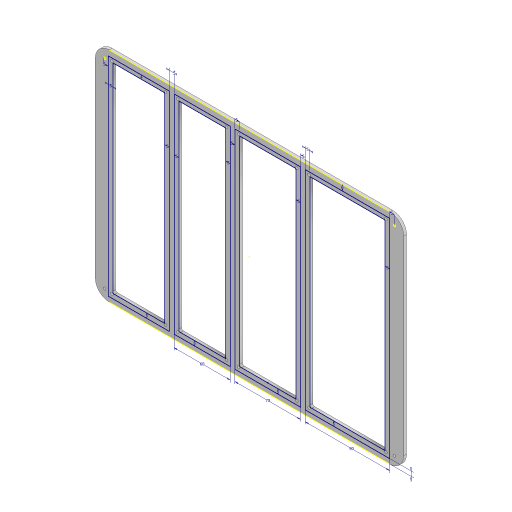
# Autodesk Inventor part: рамка насу
Saved by Autodesk Inventor 2023.2 (Build 272271000, 271)
## iProperties
Created: 2023-02-13
Part Number: рамка насу
Material: Типовые
Document SubType Name: Modeling
Designer: User
Density: 1 g/cm^3
Appearance: По умолчанию
Author: User
Autodesk Inventor part; units mm, degrees
ref_plane "YZ Plane" through (0, 0, 0) normal (1, 0, 0) x (0, 1, 0)
ref_plane "XZ Plane" through (0, 0, 0) normal (0, 1, 0) x (-1, 0, 0)
ref_plane "XY Plane" through (0, 0, 0) normal (0, 0, 1) x (1, 0, 0)
sketch "Эскиз1" plane through (0, 0, 0) normal (0, 0, 1) x (1, 0, 0)
  line L0 (-149.5, 116.5) -> (149.5, 116.5)
  line L1 (164.5, 101.5) -> (164.5, -101.5)
  line L2 (149.5, -116.5) -> (-149.5, -116.5)
  line L3 (-164.5, -101.5) -> (-164.5, 101.5)
  line L4 (0, -167.4492) -> (0, 167.4492) projected
  line L5 (-234.6492, 0) -> (234.6492, 0) projected
  arc A0 (-149.5, 116.5) -> (-164.5, 101.5) centre (-149.5, 101.5) ccw
  arc A1 (164.5, 101.5) -> (149.5, 116.5) centre (149.5, 101.5) ccw
  arc A2 (149.5, -116.5) -> (164.5, -101.5) centre (149.5, -101.5) ccw
  arc A3 (-164.5, -101.5) -> (-149.5, -116.5) centre (-149.5, -101.5) ccw
  circle A4 centre (-154.5, 106.5) radius 1.35
  circle A5 centre (154.5, 106.5) radius 1.35
  circle A6 centre (154.5, -106.5) radius 1.35
  circle A7 centre (-154.5, -106.5) radius 1.35
  point P0 (0, 0)
  dimension "d0" = 329
  dimension "d1" = 233
  dimension "d2" = 15
  dimension "d3" = 2.7
  dimension "d4" = 2.7
  dimension "d5" = 2.7
  dimension "d6" = 2.7
  dimension "d7" = 5
  dimension "d8" = 5
  dimension "d9" = 5
  dimension "d10" = 5
  dimension "d11" = 5
  dimension "d12" = 5
  dimension "d13" = 5
  dimension "d14" = 5
  constraints: 8 centre point, 8 end point, 8 point on circle, 8 tangent, 3 equal radius, 2 parallel, 1 horizontal, 1 perpendicular, 2 other
  measures "d0" distance between parallel lines of L1 L3
  measures "d1" distance between parallel lines of L2 L0
  measures "d2" radius of A0
  measures "d3" diameter of A4
  measures "d4" diameter of A5
  measures "d5" diameter of A6
  measures "d6" diameter of A7
  measures "d7" horizontal distance of A6.centre A2.centre
  measures "d8" horizontal distance of A2.centre A6.centre
  measures "d9" horizontal distance of A1.centre A5.centre
  measures "d10" horizontal distance of A5.centre A1.centre
  measures "d11" horizontal distance of A0.centre A4.centre
  measures "d12" horizontal distance of A0.centre A4.centre
  measures "d13" horizontal distance of A7.centre A3.centre
  measures "d14" horizontal distance of A3.centre A7.centre
extrude "Выдавливание1" add sketch "Эскиз1" along normal blind 3
sketch "Эскиз2" plane through (0, 0, 3) normal (0, 0, 1) x (1, 0, 0)
  line L0 (149.5, 110.5) -> (59.5, 110.5)
  line L1 (59.5, 110.5) -> (59.5, -111.5)
  line L2 (59.5, -111.5) -> (149.5, -111.5)
  line L3 (149.5, -111.5) -> (149.5, 110.5)
  line L4 (54.5, 110.5) -> (-15.5, 110.5)
  line L5 (-15.5, 110.5) -> (-15.5, -111.5)
  line L6 (-15.5, -111.5) -> (54.5, -111.5)
  line L7 (54.5, -111.5) -> (54.5, 110.5)
  line L8 (-20.5, 110.5) -> (-80.5, 110.5)
  line L9 (-80.5, 110.5) -> (-80.5, -111.5)
  line L10 (-80.5, -111.5) -> (-20.5, -111.5)
  line L11 (-20.5, -111.5) -> (-20.5, 110.5)
  circle A0 centre (154.5, 106.5) radius 1.35 projected
  line L12 (-85.5, 110.5) -> (-150.85, 110.5)
  line L13 (-150.85, 110.5) -> (-150.85, -111.5)
  line L14 (-150.85, -111.5) -> (-85.5, -111.5)
  line L15 (-85.5, -111.5) -> (-85.5, 110.5)
  circle A1 centre (-154.5, 106.5) radius 1.35 projected
  line L16 (-149.5, -116.5) -> (149.5, -116.5) projected
  line L17 (149.5, 116.5) -> (-149.5, 116.5) projected
  line L18 (-145.85, 106.5) -> (-90.5, 106.5)
  line L19 (-90.5, 106.5) -> (-90.5, -106.5)
  line L20 (-90.5, -106.5) -> (-145.85, -106.5)
  line L21 (-145.85, -106.5) -> (-145.85, 106.5)
  line L22 (-75.5, 106.5) -> (-25.5, 106.5)
  line L23 (-25.5, 106.5) -> (-25.5, -106.5)
  line L24 (-25.5, -106.5) -> (-75.5, -106.5)
  line L25 (-75.5, -106.5) -> (-75.5, 106.5)
  line L26 (-10.5, 106.5) -> (49.5, 106.5)
  line L27 (49.5, 106.5) -> (49.5, -106.5)
  line L28 (49.5, -106.5) -> (-10.5, -106.5)
  line L29 (-10.5, -106.5) -> (-10.5, 106.5)
  line L30 (64.5, 106.5) -> (144.5, 106.5)
  line L31 (144.5, 106.5) -> (144.5, -106.5)
  line L32 (144.5, -106.5) -> (64.5, -106.5)
  line L33 (64.5, -106.5) -> (64.5, 106.5)
  point P0 (0, 0)
  point P1 (19.5, -106.5)
  dimension "d18" = 70
  dimension "d19" = 60
  dimension "d20" = 5
  dimension "d21" = 5
  dimension "d22" = 5
  dimension "d23" = 90
  dimension "d25" = 5
  dimension "d26" = 5
  dimension "d27" = 5
  dimension "d29" = 6
  dimension "d30" = 4
  dimension "d31" = 5
  dimension "d32" = 5
  dimension "d33" = 5
  dimension "d34" = 5
  dimension "d35" = 5
  dimension "d36" = 5
  dimension "d37" = 5
  dimension "d38" = 5
  dimension "d39" = 5
  dimension "d40" = 5
  dimension "d41" = 5
  dimension "d42" = 5
  constraints: 64 end point, 16 parallel, 8 horizontal, 8 perpendicular, 5 horizontal alignment, 4 point on line, 1 midpoint
  measures "d18" distance of L6.end L5.end
  measures "d19" distance of L10.end L9.end
  measures "d20" distance between parallel lines of L7 L1
  measures "d21" distance from line of A0.centre L3
  measures "d22" distance between parallel lines of L11 L5
  measures "d23" distance between parallel lines of L3 L1
  measures "d25" distance between parallel lines of L15 L9
  measures "d27" distance between parallel lines of L2 L16
  measures "d29" distance between parallel lines of L17 L0
  measures "d30" distance between parallel lines of L12 L18
  measures "d31" distance between parallel lines of L15 L19
  measures "d32" distance between parallel lines of L13 L21
  measures "d33" distance between parallel lines of L14 L20
  measures "d34" distance between parallel lines of L1 L33
  measures "d35" distance between parallel lines of L31 L3
  measures "d36" distance between parallel lines of L2 L32
  measures "d37" distance between parallel lines of L5 L29
  measures "d38" distance between parallel lines of L7 L27
  measures "d39" distance from line of L6 point (19.5, -106.5)
  measures "d40" distance between parallel lines of L9 L25
  measures "d41" distance between parallel lines of L11 L23
  measures "d42" distance between parallel lines of L10 L24
extrude "Выдавливание2" cut sketch "Эскиз2" against normal blind 3 contours L18 L19 L20 L21 | L22 L23 L24 L25 | L26 L27 L28 L29 | L30 L31 L32 L33
sketch "Эскиз3" plane through (0, 0, 3) normal (0, 0, 1) x (1, 0, 0)
  circle A0 centre (-146.85, 107.5) radius 1.35
  circle A1 centre (-89.5, 107.5) radius 1.35
  circle A2 centre (-146.85, -107.5) radius 1.35
  circle A3 centre (-89.5, -107.5) radius 1.35
  line L0 (-145.85, -106.5) -> (-145.85, 106.5) projected
  line L1 (-145.85, 106.5) -> (-90.5, 106.5) projected
  line L2 (-90.5, 106.5) -> (-90.5, -106.5) projected
  line L3 (-90.5, -106.5) -> (-145.85, -106.5) projected
  circle A4 centre (-76.5, -107.5) radius 1.35
  circle A5 centre (-24.5, -107.5) radius 1.35
  circle A6 centre (-76.5, 107.5) radius 1.35
  circle A7 centre (-24.5, 107.5) radius 1.35
  circle A8 centre (-11.5, 107.5) radius 1.35
  circle A9 centre (-11.5, -107.5) radius 1.35
  circle A10 centre (50.5, -107.5) radius 1.35
  circle A11 centre (50.5, 107.5) radius 1.35
  line L4 (-75.5, -106.5) -> (-75.5, 106.5) projected
  line L5 (-75.5, 106.5) -> (-25.5, 106.5) projected
  line L6 (-25.5, 106.5) -> (-25.5, -106.5) projected
  line L7 (-25.5, -106.5) -> (-75.5, -106.5) projected
  line L8 (-10.5, -106.5) -> (-10.5, 106.5) projected
  line L9 (-10.5, 106.5) -> (49.5, 106.5) projected
  line L10 (49.5, 106.5) -> (49.5, -106.5) projected
  line L11 (49.5, -106.5) -> (-10.5, -106.5) projected
  circle A12 centre (63.5, 107.5) radius 1.35
  circle A13 centre (63.5, -107.5) radius 1.35
  circle A14 centre (145.5, -107.5) radius 1.35
  circle A15 centre (145.5, 107.5) radius 1.35
  line L12 (64.5, -106.5) -> (64.5, 106.5) projected
  line L13 (64.5, 106.5) -> (144.5, 106.5) projected
  line L14 (144.5, 106.5) -> (144.5, -106.5) projected
  line L15 (144.5, -106.5) -> (64.5, -106.5) projected
  point P0 (0, 0)
  dimension "d45" = 2.7
  dimension "d46" = 2.7
  dimension "d47" = 2.7
  dimension "d48" = 2.7
  dimension "d49" = 1
  dimension "d51" = 1
  dimension "d52" = 1
  dimension "d53" = 1
  dimension "d54" = 1
  dimension "d55" = 1
  dimension "d56" = 1
  dimension "d57" = 1
  dimension "d58" = 2.7
  dimension "d59" = 2.7
  dimension "d60" = 2.7
  dimension "d61" = 2.7
  dimension "d62" = 2.7
  dimension "d63" = 2.7
  dimension "d64" = 2.7
  dimension "d65" = 2.7
  dimension "d66" = 1
  dimension "d67" = 1
  dimension "d68" = 1
  dimension "d69" = 1
  dimension "d70" = 1
  dimension "d71" = 1
  dimension "d72" = 1
  dimension "d73" = 1
  dimension "d74" = 1
  dimension "d75" = 1
  dimension "d76" = 1
  dimension "d77" = 1
  dimension "d78" = 1
  dimension "d79" = 1
  dimension "d80" = 1
  dimension "d81" = 1
  dimension "d82" = 2.7
  dimension "d83" = 2.7
  dimension "d84" = 2.7
  dimension "d85" = 2.7
  dimension "d86" = 1
  dimension "d87" = 1
  dimension "d88" = 1
  dimension "d89" = 1
  dimension "d90" = 1
  dimension "d91" = 1
  dimension "d92" = 1
  dimension "d93" = 1
  constraints: 16 centre point
  measures "d45" diameter of A0
  measures "d46" diameter of A1
  measures "d47" diameter of A2
  measures "d48" diameter of A3
  measures "d49" distance from line of L0 A0.centre
  measures "d51" distance from line of L1 A0.centre
  measures "d52" distance from line of L2 A1.centre
  measures "d53" distance from line of L1 A1.centre
  measures "d54" distance from line of A3.centre L3
  measures "d55" distance from line of L2 A3.centre
  measures "d56" distance from line of L0 A2.centre
  measures "d57" distance from line of L3 A2.centre
  measures "d58" diameter of A4
  measures "d59" diameter of A5
  measures "d60" diameter of A6
  measures "d61" diameter of A7
  measures "d62" diameter of A8
  measures "d63" diameter of A9
  measures "d64" diameter of A10
  measures "d65" diameter of A11
  measures "d66" distance from line of L4 A6.centre
  measures "d67" distance from line of L5 A6.centre
  measures "d68" distance from line of L5 A7.centre
  measures "d69" distance from line of L6 A7.centre
  measures "d70" distance from line of L7 A4.centre
  measures "d71" distance from line of A4.centre L4
  measures "d72" distance from line of L7 A5.centre
  measures "d73" distance from line of L6 A5.centre
  measures "d74" distance from line of L8 A8.centre
  measures "d75" distance from line of L9 A8.centre
  measures "d76" distance from line of L9 A11.centre
  measures "d77" distance from line of L10 A11.centre
  measures "d78" distance from line of L11 A9.centre
  measures "d79" distance from line of L8 A9.centre
  measures "d80" distance from line of L11 A10.centre
  measures "d81" distance from line of L10 A10.centre
  measures "d82" diameter of A12
  measures "d83" diameter of A13
  measures "d84" diameter of A14
  measures "d85" diameter of A15
  measures "d86" distance from line of L12 A12.centre
  measures "d87" distance from line of L13 A12.centre
  measures "d88" distance from line of L14 A15.centre
  measures "d89" distance from line of L13 A15.centre
  measures "d90" distance from line of L15 A14.centre
  measures "d91" distance from line of L14 A14.centre
  measures "d92" distance from line of L12 A13.centre
  measures "d93" distance from line of L15 A13.centre
extrude "Выдавливание3" cut sketch "Эскиз3" against normal blind 10 contours A0 | A1 | A2 | A3 | A4 | A5 | A6 | A7 | A8 | A9 | A10 | A11 | A12 | A13 | A14 | A15
fillet "Сопряжение1" radius 2 1 edges at (64.5, 106.5, 1.5)
fillet "Сопряжение2" radius 2 5 edges at (144.5, 106.5, 1.5) (64.5, -106.5, 1.5) (144.5, -106.5, 1.5) (49.5, -106.5, 1.5) (-10.5, -106.5, 1.5)
fillet "Сопряжение3" radius 2 6 edges at (-10.5, 106.5, 1.5) (49.5, 106.5, 1.5) (-25.5, 106.5, 1.5) (-75.5, 106.5, 1.5) (-25.5, -106.5, 1.5) (-75.5, -106.5, 1.5)
fillet "Сопряжение4" radius 2 4 edges at (-145.85, -106.5, 1.5) (-90.5, -106.5, 1.5) (-90.5, 106.5, 1.5) (-145.85, 106.5, 1.5)
